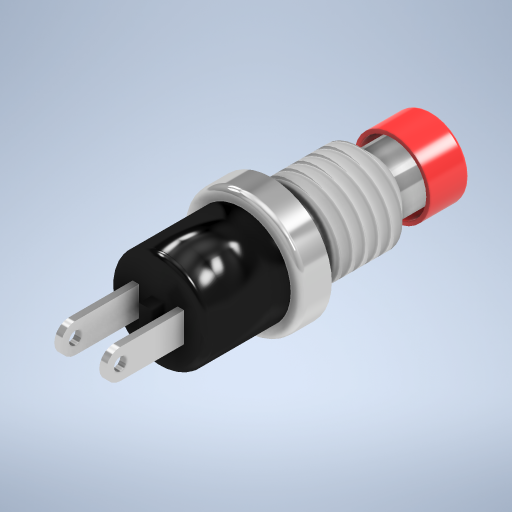
# Autodesk Inventor part: BUTTON
Saved by Autodesk Inventor 2023 (Build 270158000, 158)
## iProperties
Created: 2023-03-15
Part Number: BUTTON
Material: Generic
Document SubType Name: Modeling
Designer: Amos Yu
Density: 1 g/cm^3
Appearance: Default
Author: Amos Yu
Autodesk Inventor part; units mm, degrees
ref_plane "XZ Plane" through (0, 0, 0) normal (0, 1, 0) x (-1, 0, 0)
ref_plane "XY Plane" through (0, 0, 0) normal (0, 0, 1) x (1, 0, 0)
sketch "Sketch1" plane through (0, 0, 0) normal (0, 1, 0) x (-1, 0, 0)
  line L0 (0, 0) -> (0, -21.3)
  line L1 (0, 0) -> (3.3, 0)
  line L2 (3.8, -0.5) -> (3.8, -6.5)
  line L3 (3.8, -6.5) -> (4.2, -6.5)
  line L4 (4.7, -7) -> (4.7, -8.8)
  line L5 (4.7, -8.8) -> (2.9, -8.8)
  line L6 (2.9, -8.8) -> (2.9, -10.2)
  line L7 (2.9, -10.2) -> (3.4, -10.2)
  line L8 (3.4, -10.2) -> (3.4, -15.6)
  line L9 (3.4, -15.6) -> (2.3, -16.7)
  line L10 (2.3, -16.7) -> (2.3, -21)
  arc A0 (3.8, -0.5) -> (3.3, 0) centre (3.3, -0.5) ccw
  arc A1 (4.7, -7) -> (4.2, -6.5) centre (4.2, -7) ccw
  line L11 (2.3, -21) -> (2.65, -21)
  line L12 (2.65, -21) -> (2.65, -18.2)
  line L13 (2.65, -18.2) -> (2.95, -18.2)
  line L14 (2.95, -18.2) -> (2.95, -21)
  line L15 (2.65, -21.3) -> (0, -21.3)
  arc A2 (2.65, -21.3) -> (2.95, -21) centre (2.65, -21) ccw
  point P0 (3.8, 0)
  point P1 (4.7, -6.5)
  point P2 (2.95, -21.3)
  dimension "d0" = 7.6
  dimension "d1" = 9.4
  dimension "d2" = 5.8
  dimension "d3" = 6.8
  dimension "d4" = 4.6
  dimension "d5" = 2.3
  dimension "d6" = 8.8
  dimension "d7" = 1.4
  dimension "d8" = 5.4
  dimension "d9" = 135
  dimension "d11" = 0.5
  dimension "d12" = 21.3
  dimension "d13" = 0.3
  dimension "d14" = 0.3
  dimension "d15" = 5.9
  dimension "d16" = 3.1
  dimension "d18" = 0.3
  constraints: 32 end point, 10 perpendicular, 6 point on circle, 6 point on line, 6 tangent, 3 centre point, 3 horizontal, 1 equal radius, 1 parallel, 1 vertical
  measures "d0" diameter of L2 L0
  measures "d1" diameter of L4 L0
  measures "d2" diameter of L6 L0
  measures "d3" diameter of L8 L0
  measures "d4" diameter of L10 L0
  measures "d5" distance of point (4.7, -6.5) L4.end
  measures "d6" vertical distance of L4.end point (3.8, 0)
  measures "d7" distance of L5.end L6.end
  measures "d8" distance of L7.end L8.end
  measures "d9" angle of L8 L9
  measures "d11" radius of A0
  measures "d12" distance of L0.start L0.end
  measures "d13" distance between parallel lines of L15 L11
  measures "d14" distance between parallel lines of L14 L12
  measures "d15" diameter of L14 L0
  measures "d16" distance of L13.end point (2.95, -21.3)
  measures "d18" radius of A2
revolve "Revolution1" add sketch "Sketch1" angle 360 about axis through (0, 0, 0) along (0, 0, -1)
thread "Thread1" size "M7x1" class "6g" standard "ANSI Metric M Profile" full length
ref_plane "Work Plane1" through (1.5, 0, 0) normal (1, 0, 0) x (0, 1, 0)
sketch "Sketch2" plane through (1.5, 0, 0) normal (1, 0, 0) x (0, 1, 0)
  line L0 (-1.15, 4.95) -> (-1.15, 0)
  line L1 (-1.15, 0) -> (1.15, 0)
  line L2 (1.15, 0) -> (1.15, 4.95)
  arc A0 (1.15, 4.95) -> (-1.15, 4.95) centre (0, 4.95) ccw
  circle A1 centre (0, 4.95) radius 0.5
  point P0 (0, 0)
  point P1 (0, 0)
  dimension "d22" = 2.3
  dimension "d23" = 4.95
  dimension "d24" = 1
  constraints: 6 end point, 2 centre point, 2 coincident, 2 point on circle, 2 tangent, 1 horizontal, 1 midpoint, 1 parallel, 1 perpendicular
  measures "d22" distance of L1.end L0.end
  measures "d23" distance of L0.end L0.start
  measures "d24" diameter of A1
extrude "Extrusion1" add sketch "Sketch2" along normal blind 0.5
mirror "Mirror1" about plane through (0, 0, 0) normal (1, 0, 0) of "Extrusion1"
sketch "Sketch3" plane through (0, 0, 0) normal (0, 0, 1) x (1, 0, 0)
  line L0 (-0.5, 0.9) -> (0.5, 0.9)
  line L1 (0.5, 0.9) -> (0.5, -0.9)
  line L2 (0.5, -0.9) -> (-0.5, -0.9)
  line L3 (-0.5, -0.9) -> (-0.5, 0.9)
  line L4 (-0.5, -0.9) -> (0.5, 0.9) construction
  line L5 (-0.5, 0.9) -> (0.5, -0.9) construction
  point P0 (0, 0)
  point P1 (0, 0)
  dimension "d27" = 1
  dimension "d28" = 1.8
  constraints: 12 end point, 2 parallel, 1 coincident, 1 horizontal, 1 midpoint, 1 perpendicular
  measures "d27" distance of L1.end L2.end
  measures "d28" distance of L0.end L1.end
extrude "Extrusion2" add sketch "Sketch3" along normal blind 1
body "Solid1"
